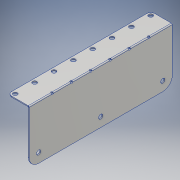
# Autodesk Inventor part: gpu_holder
Saved by Autodesk Inventor 2018 (Build 220112000, 112)
## iProperties
Created: 2019-10-14
Part Number: gpu_holder
Material: アルミニウム 6061
Document SubType Name: Sheet Metal
Designer: gisen
Density: 2.7 g/cm^3
Sheet Metal Rule: Default_mm
Appearance: アルミニウム - フラット
Sheet Metal Width: 0.000 mm
Sheet Metal Length: 0.000 mm
Sheet Metal Area: 0.000 mm^2
Author: gisen
Autodesk Inventor part; units mm, degrees
ref_plane "YZ Plane" through (0, 0, 0) normal (1, 0, 0) x (0, 1, 0)
ref_plane "XZ Plane" through (0, 0, 0) normal (0, 1, 0) x (-1, 0, 0)
ref_plane "XY Plane" through (0, 0, 0) normal (0, 0, 1) x (1, 0, 0)
sketch "スケッチ1" plane through (0, 0, 0) normal (0, 0, 1) x (1, 0, 0)
  line L0 (4, 0) -> (21.777, 0)
  line L1 (21.777, 0) -> (21.777, 151.5)
  line L2 (21.777, 151.5) -> (4, 151.5)
  line L3 (0, 147.5) -> (0, 4)
  circle A0 centre (4, 147.5) radius 2.25
  circle A1 centre (4, 127) radius 2.25
  circle A2 centre (4, 106.5) radius 2.25
  circle A3 centre (4, 86) radius 2.25
  circle A4 centre (4, 65.5) radius 2.25
  circle A5 centre (4, 45) radius 2.25
  circle A6 centre (4, 24.5) radius 2.25
  circle A7 centre (4, 4) radius 2.25
  arc A8 (4, 151.5) -> (0, 147.5) centre (4, 147.5) ccw
  arc A9 (0, 4) -> (4, 0) centre (4, 4) ccw
  point P0 (0, 0)
  point P1 (0, 151.5)
  dimension "d0" = 151.5
  dimension "d1" = 21.777
  dimension "d2" = 4.5
  dimension "d3" = 4
  dimension "d4" = 4
  dimension "d7" = 20.5
  dimension "d12" = 4
  measures "d0" distance of point (0, 151.5) point (0, 0)
  measures "d1" distance of L1.end point (0, 151.5)
  measures "d2" diameter of A0
  measures "d3" distance from line of L3 A0.centre
  measures "d4" distance from line of A0.centre L2
  measures "d7" distance of A0.centre A1.centre
  measures "d12" radius of A8
extrude "プレート1" add sketch "スケッチ1" along normal blind 1
sketch "スケッチ2" plane through (21.778, 0, -0.001) normal (1, 0, 0) x (0, 1, 0)
  line L0 (151.5, 0) -> (0, 0)
  line L1 (0, 0) -> (0, -56.366)
  line L2 (0, -56.366) -> (151.5, -56.366)
  line L3 (151.5, -56.366) -> (151.5, 0)
  constraints: 6 end point, 1 horizontal, 1 perpendicular, 1 vertical
edge flange "フランジ1" height 56.367 angle 90 thickness 1 bend radius 0 thickness toward (1, 0, 0) relief straight relief width 1 relief depth 0.5 edges at (21.777, 75.75, 0) wall of the first edge with corners at (21.778, 151.5, -0.001) (21.778, 0, -0.001) (21.778, 0, -56.367) (21.778, 151.5, -56.367)
bend "曲げ1"
corner "コーナー1"
sketch "スケッチ3" plane through (22.778, 0, -56.367) normal (1, 0, 0) x (0, 0, -1)
  circle A0 centre (-10, 141.5) radius 2.25
  circle A1 centre (-10, 10) radius 2.25
  line L0 (0, 151.5) -> (0, 0) projected
  line L1 (-56.366, 151.5) -> (0, 151.5) projected
  line L2 (0, 0) -> (-56.366, 0) projected
  line L3 (-10, 10) -> (-10, 141.5) construction
  circle A2 centre (-10, 75.75) radius 2.25
  point P0 (-56.367, 0)
  dimension "d24" = 4.5
  dimension "d25" = 10
  dimension "d26" = 10
  dimension "d27" = 10
  dimension "d28" = 10
  constraints: 3 centre point, 2 end point, 2 equal radius, 1 midpoint
  measures "d24" diameter of A0
  measures "d25" distance from line of L0 L3.end
  measures "d26" distance from line of L0 L3.start
  measures "d27" distance from line of L3.end L1
  measures "d28" distance from line of L2 L3.start
extrude "押し出し1" cut sketch "スケッチ3" against normal blind 1
fillet "フィレット1" radius 10 2 edges at (22.278, 151.5, -56.367) (22.278, 0, -56.367)
unfold all bends "展開1" k factor 0.44 fixed face at (16.602, 72.3333, 1)
sketch "スケッチ4" plane through (78.8357, 10, 1) normal (0, 0, 1) x (1, 0, 0)
  line L0 (-56.366, 141.5) -> (-56.366, -10) construction
  line L1 (-57.0587, 141.5) -> (-56.366, 141.5) construction
  line L2 (-57.0587, 141.5) -> (-57.0587, -10) construction
  line L3 (-56.366, -10) -> (-57.0587, -10) construction
  line L4 (-56.7124, -10) -> (-56.7124, 141.5) construction
  line L5 (-57.0587, 141.5) -> (-56.366, 141.5) projected
  circle A0 centre (-74.8357, -6) radius 2.25 construction
  circle A1 centre (-74.8357, 14.5) radius 2.25 construction
  circle A2 centre (-74.8357, 35) radius 2.25 construction
  circle A3 centre (-74.8357, 55.5) radius 2.25 construction
  circle A4 centre (-74.8357, 76) radius 2.25 construction
  circle A5 centre (-74.8357, 96.5) radius 2.25 construction
  circle A6 centre (-74.8357, 117) radius 2.25 construction
  circle A7 centre (-74.8357, 137.5) radius 2.25 construction
  line L6 (-74.8357, -6) -> (-56.7124, -6) construction
  line L7 (-74.8357, 14.5) -> (-56.7124, 14.5) construction
  circle A8 centre (-74.8357, 35) radius 2.25 construction
  line L8 (-74.8357, 35) -> (-56.7124, 35) construction
  line L9 (-74.8357, 55.5) -> (-56.7124, 55.5) construction
  line L10 (-74.8357, 76) -> (-56.7124, 76) construction
  line L11 (-74.8357, 96.5) -> (-56.7124, 96.5) construction
  line L12 (-74.8357, 117) -> (-56.7124, 117) construction
  circle A9 centre (-74.8357, 137.5) radius 2.25 construction
  line L13 (-74.8357, 137.5) -> (-56.7124, 137.5) construction
  circle A10 centre (-56.7124, 14.5) radius 1.05
  circle A11 centre (-56.7124, 117) radius 1.05
  circle A12 centre (-56.7124, 55.5) radius 1.05
  circle A13 centre (-56.7124, 76) radius 1.05
  circle A14 centre (-56.7124, 35) radius 1.05
  circle A15 centre (-56.7124, 96.5) radius 1.05
  point P0 (-78.8357, -10)
  dimension "d32" = 2.1
  constraints: 16 end point, 7 horizontal, 6 centre point, 6 coincident, 5 equal radius, 2 midpoint, 1 parallel, 11 other
  measures "d32" diameter of A10
extrude "押し出し2" cut sketch "スケッチ4" against normal up to surface (1 mm away)
refold all bends "再折り曲げ1"
equation "\"d26\" = d25"
equation "\"d28\" = d27"
equation "\"d29\" = Thickness"
equation "\"d13\" = Thickness"
equation "\"d14\" = BendReliefWidth"
equation "\"d15\" = BendReliefDepth"
equation "\"d16\" = MinimumRemnant"
equation "\"d21\" = CornerReliefSize"
equation "\"d22\" = GapSize"
equation "\"BendReliefWidth\" = Thickness"
equation "\"BendReliefDepth\" = 0.5 * Thickness"
equation "\"CornerReliefSize\" = 4 * Thickness"
equation "\"MinimumRemnant\" = 2 * Thickness"
equation "\"GapSize\" = Thickness"
equation "\"Thickness\" = 1"
